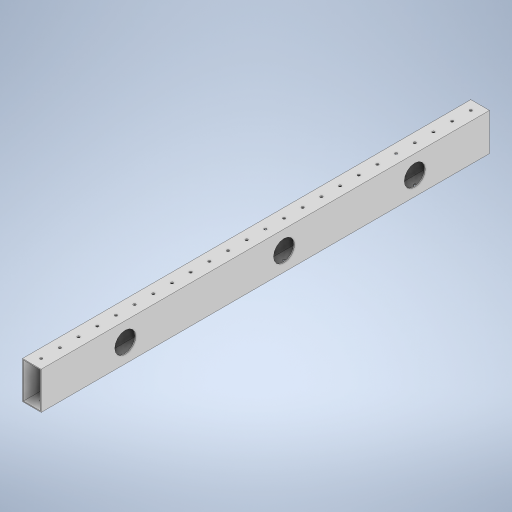
# Autodesk Inventor part: intake versa
Saved by Autodesk Inventor 2023.2 (Build 272271000, 271)
## iProperties
Created: 2020-01-13
Part Number: intake versa
Material: Generic
Document SubType Name: Modeling
Designer: aidan
Density: 1 g/cm^3
Appearance: Default
Author: aidan
Autodesk Inventor part; units mm, degrees
ref_plane "YZ Plane" through (0, 0, 0) normal (1, 0, 0) x (0, 1, 0)
ref_plane "XZ Plane" through (0, 0, 0) normal (0, 1, 0) x (-1, 0, 0)
ref_plane "XY Plane" through (0, 0, 0) normal (0, 0, 1) x (1, 0, 0)
sketch "Sketch1" plane through (0, 0, 0) normal (0, 0, 1) x (1, 0, 0)
  line L0 (-12.1708, 16.0073) -> (13.2292, 16.0073)
  line L1 (13.2292, 16.0073) -> (13.2292, -34.7927)
  line L2 (13.2292, -34.7927) -> (-12.1708, -34.7927)
  line L3 (-12.1708, -34.7927) -> (-12.1708, 16.0073)
  line L4 (11.9592, 14.7373) -> (-10.9008, 14.7373)
  line L5 (-10.9008, 14.7373) -> (-10.9008, -33.5227)
  line L6 (-10.9008, -33.5227) -> (11.9592, -33.5227)
  line L7 (11.9592, -33.5227) -> (11.9592, 14.7373)
  point P0 (0, 0)
  dimension "d0" = 25.4
  dimension "d1" = 50.8
  dimension "d2" = 1.27
  constraints: 16 end point, 4 parallel, 2 perpendicular, 1 horizontal, 3 other
  measures "d0" distance of L0.start L0.end
  measures "d1" distance of L0.end L1.end
  measures "d2" distance between parallel lines of L0 L4
extrude "Extrusion1" add sketch "Sketch1" along normal blind 609.6
sketch "Sketch2" plane through (-12.1708, 16.0073, 0) normal (0, 1, 0) x (1, 0, 0)
  circle A0 centre (12.7, -12.7) radius 1.7272
  line L0 (25.4, 0) -> (0, 0) projected
  line L1 (0, 0) -> (0, -609.6) projected
  point P0 (12.1708, 0)
  dimension "d5" = 3.4544
  dimension "d6" = 12.7
  dimension "d7" = 12.7
  constraints: 1 centre point
  measures "d5" diameter of A0
  measures "d6" distance from line of L0 A0.centre
  measures "d7" distance from line of L1 A0.centre
extrude "Extrusion2" cut sketch "Sketch2" against normal through all
pattern_linear "Rectangular Pattern1" count 61 spacing 25.4 along (0, 0, 1) of "Extrusion2"
sketch "Sketch3" plane through (13.2292, -34.7927, 0) normal (1, 0, 0) x (0, 0, -1)
  circle A0 centre (-495.3, 25.4) radius 14.2875
  line L0 (-609.6, 0) -> (-609.6, 50.8) projected
  line L1 (0, 0) -> (-609.6, 0) projected
  circle A1 centre (-279.4, 25.4) radius 14.2875
  circle A2 centre (-101.6, 25.4) radius 14.2875
  point P0 (0, 34.7927)
  point P1 (-609.6, 25.4)
  dimension "d15" = 28.575
  dimension "d16" = 114.3
  dimension "d17" = 25.4
  dimension "d18" = 28.575
  dimension "d19" = 330.2
  dimension "d20" = 28.575
  dimension "d21" = 177.8
  dimension "d22" = 25.4
  dimension "d23" = 25.4
  constraints: 3 centre point, 1 midpoint
  measures "d15" diameter of A0
  measures "d16" distance from line of A0.centre L0
  measures "d17" distance from line of L1 A0.centre
  measures "d18" diameter of A1
  measures "d19" distance of A1.centre point (-609.6, 25.4)
  measures "d20" diameter of A2
  measures "d21" distance of A1.centre A2.centre
  measures "d22" distance from line of L1 A2.centre
  measures "d23" distance from line of L1 A1.centre
extrude "Extrusion3" cut sketch "Sketch3" against normal blind 214.3125
equation "\"d3\" = d13"
equation "\"d10\" = d14"
equation "\"d13\" = 609.6"
equation "\"d14\" = d13"
body "Solid1"
